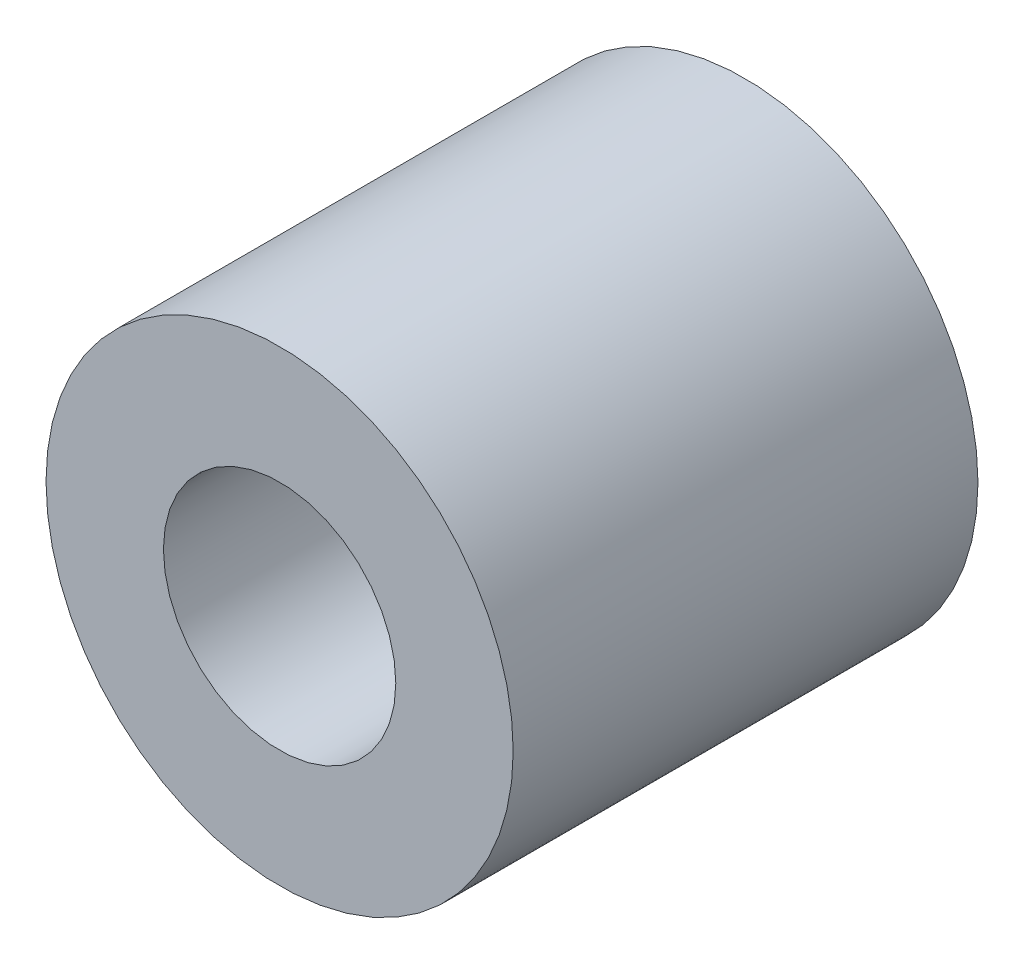
# Autodesk Inventor part: TrapLimiter
Saved by Autodesk Inventor 2019 (Build 230136000, 136)
## iProperties
Created: 2018-12-18
Part Number: TrapLimiter
Material: Generic
Document SubType Name: Modeling
Designer: assman
Density: 1 g/cm^3
Appearance: Default
Author: assman
Autodesk Inventor part; units mm, degrees
ref_plane "YZ Plane" through (0, 0, 0) normal (1, 0, 0) x (0, 1, 0)
ref_plane "XZ Plane" through (0, 0, 0) normal (0, 1, 0) x (-1, 0, 0)
ref_plane "XY Plane" through (0, 0, 0) normal (0, 0, 1) x (1, 0, 0)
ref_plane "Work Plane1" through (0, 0, 0) normal (0, 0, 1) x (1, 0, 0)
sketch "Sketch1" plane through (0, 0, 0) normal (0, 0, 1) x (1, 0, 0)
  circle A0 centre (35.2586, -12.6608) radius 2.0105 construction
  circle A1 centre (35.2586, -12.6608) radius 2.0105
  point P0 (0, 0)
  dimension "d1" = 4.021
  constraints: 2 centre point, 2 coincident, 1 concentric
  measures "d1" diameter of A0
extrude "Extrusion1" add sketch "Sketch1" along normal blind 4
sketch "Sketch2" plane through (35.2586, -12.6608, 4) normal (0, 0, 1) x (1, 0, 0)
  circle A0 centre (0, 0) radius 2.0105 projected
  point P0 (-35.2586, 12.6608)
  constraints: 1 coincident
hole "Hole1" at (35.2586, -12.6608, 4) direction (0, 0, -1) diameter 2 end through all
body "Solid1"
